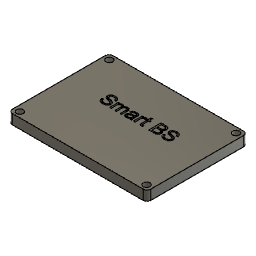
SmartEFM_BS_TopCover_@ v4 (Autodesk Fusion 360 design; units mm, degrees)
Autodesk Fusion 360 part; units mm, degrees
sketch "Sketch1" plane through (0, 0, 0) normal (0, 1, 0) x (1, 0, 0)
  line L0 (0, 0) -> (113, 0)
  line L1 (113, 0) -> (113, -82)
  line L2 (113, -82) -> (0, -82)
  line L3 (0, -82) -> (0, 0)
  dimension "d1" = 113
  dimension "d2" = 82
  constraint horizontal L0
  constraint vertical L1
  constraint horizontal L2
  constraint vertical L3
  constraint coincident L0.start L3.end
  measures "d1" distance of L0.start L0.end
  measures "d2" distance of L0.start L2.end
extrude "Extrude1" add sketch "Sketch1" along normal blind 8
fillet "Fillet1" radius 3 4 edges at (0, 4, 82) (113, 4, 82) (113, 4, 0) (0, 4, 0)
sketch "Sketch2" plane through (0, 8, 0) normal (0, 1, 0) x (-1, 0, 0)
  arc A0 (-3, 0) -> (0, 3) centre (-3, 3) ccw
  line L0 (0, 3) -> (0, 79)
  arc A1 (0, 79) -> (-3, 82) centre (-3, 79) ccw
  line L1 (-3, 82) -> (-110, 82)
  arc A2 (-110, 82) -> (-113, 79) centre (-110, 79) ccw
  line L2 (-113, 79) -> (-113, 3)
  arc A3 (-113, 3) -> (-110, 0) centre (-110, 3) ccw
  line L3 (-110, 0) -> (-3, 0)
  circle A4 centre (-4.7859, 4.4507) radius 2.75
  line L4 (0, 41) -> (-113, 41)
  line L5 (-56.5, 82) -> (-56.5, 0)
  circle A5 centre (-4.7859, 77.5493) radius 2.75
  circle A6 centre (-108.2141, 4.4507) radius 2.75
  circle A7 centre (-108.2141, 77.5493) radius 2.75
  dimension "d7" = 5.5
  constraint midpoint L0 L4.start
  constraint midpoint L2 L4.end
  constraint midpoint L1 L5.start
  constraint midpoint L3 L5.end
  constraint symmetric A4 L4 A5
  constraint symmetric A4 L5 A6
  constraint symmetric L4 A6 A7
  measures "d7" diameter of A4
extrude "Extrude2" cut sketch "Sketch2" against normal blind 9 contours A4 | A5 | A6 | A7
sketch "Sketch3" plane through (0, 8, 0) normal (0, 1, 0) x (-1, 0, 0)
  circle A0 centre (-108.2141, 4.4507) radius 2.75
  circle A1 centre (-4.7859, 4.4507) radius 2.75
  circle A2 centre (-108.2141, 77.5493) radius 2.75
  circle A3 centre (-4.7859, 77.5493) radius 2.75
  arc A4 (-3, 0) -> (0, 3) centre (-3, 3) ccw
  line L0 (0, 3) -> (0, 79)
  arc A5 (0, 79) -> (-3, 82) centre (-3, 79) ccw
  line L1 (-3, 82) -> (-110, 82)
  arc A6 (-110, 82) -> (-113, 79) centre (-110, 79) ccw
  line L2 (-113, 79) -> (-113, 3)
  arc A7 (-113, 3) -> (-110, 0) centre (-110, 3) ccw
  line L3 (-110, 0) -> (-3, 0)
  line L4 (-28.8596, 42.924) -> (-88.8596, 42.924) construction
  line L5 (-88.8596, 42.924) -> (-88.8596, 27.924) construction
  line L6 (-88.8596, 27.924) -> (-28.8596, 27.924) construction
  line L7 (-28.8596, 27.924) -> (-28.8596, 42.924) construction
  dimension "d10" = 10
  text T0 "Smart BS" font "Arial" height 10 align left top in box 60 x 15 at (-28.8596, 42.924) x (-1, 0) y (0, -1) spacing 1
extrude "Extrude3" cut sketch "Sketch3" against normal blind 3 text T0
